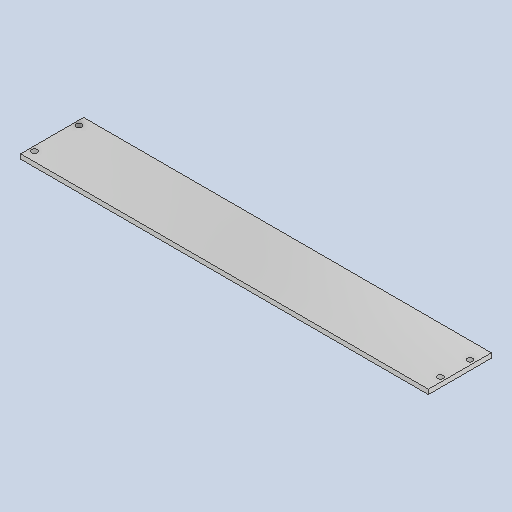
# Autodesk Inventor part: AR-Bracket(middle)2
Saved by Autodesk Inventor 2025.1 (Build 291241020, 241B)
## iProperties
Created: 2025-01-21
Part Number: AR-Bracket(middle)2
Material: Generic
Document SubType Name: Modeling
Designer: Sven
Density: 1 g/cm^3
Appearance: Aluminum - Polished
Author: Sven
Autodesk Inventor part; units mm, degrees
ref_plane "YZ Plane" through (0, 0, 0) normal (1, 0, 0) x (0, 1, 0)
ref_plane "XZ Plane" through (0, 0, 0) normal (0, 1, 0) x (-1, 0, 0)
ref_plane "XY Plane" through (0, 0, 0) normal (0, 0, 1) x (1, 0, 0)
sketch "Sketch10" plane through (0, 0, 0) normal (0, 1, 0) x (-1, 0, 0)
  line L0 (-139.7, 0) -> (-139.7, 43.18)
  line L1 (-139.7, 43.18) -> (139.7, 43.18)
  line L2 (139.7, 43.18) -> (139.7, 0)
  line L3 (139.7, 0) -> (-139.7, 0)
  point P0 (0, 0)
  point P1 (0, 0)
  dimension "d48" = 279.4
  dimension "d49" = 43.18
  dimension "d51" = 139.7
  constraints: 8 end point, 1 coincident, 1 horizontal, 1 midpoint, 1 parallel, 1 perpendicular
  measures "d48" distance of L0.end L1.end
  measures "d49" distance between parallel lines of L1 L3
  measures "d51" distance from line of point (0, 0) L0
extrude "Extrusion8" add sketch "Sketch10" along normal blind 3.175
sketch "Sketch11" plane through (0, 3.175, 0) normal (0, 1, 0) x (1, 0, 0)
  line L0 (139.7, -43.18) -> (-139.7, -43.18)
  line L1 (139.7, 0) -> (139.7, -43.18)
  line L2 (139.7, 0) -> (-139.7, 0)
  line L3 (-139.7, 0) -> (-139.7, -43.18)
  line L4 (-139.7, 0) -> (-139.7, -43.18) projected
  line L5 (-139.7, -43.18) -> (139.7, -43.18) projected
  line L6 (139.7, -43.18) -> (139.7, 0) projected
  line L7 (139.7, 0) -> (-139.7, 0) projected
  line L8 (139.7, -43.18) -> (139.7, 0) projected
  point P0 (0, 0)
  point P1 (136.525, -31.75)
  point P2 (136.525, -11.43)
  point P3 (-136.525, -6.35)
  point P4 (-136.525, -36.83)
  dimension "d54" = 11.43
  dimension "d55" = 3.175
  dimension "d56" = 11.43
  dimension "d57" = 3.175
  dimension "d58" = 3.175
  dimension "d59" = 3.175
  dimension "d60" = 6.35
  dimension "d61" = 6.35
  constraints: 8 end point, 4 collinear
  measures "d54" distance from line of L0 point (136.525, -31.75)
  measures "d55" distance from line of L1 point (136.525, -31.75)
  measures "d56" distance from line of L2 point (136.525, -11.43)
  measures "d57" distance from line of L1 point (136.525, -11.43)
  measures "d58" distance from line of point (-136.525, -36.83) L3
  measures "d59" distance from line of L3 point (-136.525, -6.35)
  measures "d60" distance from line of point (-136.525, -6.35) L2
  measures "d61" distance from line of L0 point (-136.525, -36.83)
hole "Hole2" at (-136.525, 3.175, 36.83) at (-136.525, 3.175, 6.35) at (136.525, 3.175, 11.43) at (136.525, 3.175, 31.75) direction (0, -1, 0) diameter 3.81 end through all clearance for "Flat Head Machine Screw (82)" size "#6" standard "Ansi Unified Screw Threads"
equation "\"d51\" = 0.5 * d48"
body "Solid1"
